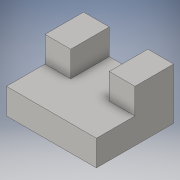
# Autodesk Inventor part: Figure 7_27_4
Saved by Autodesk Inventor 2016 (Build 200138000, 138)
## iProperties
Created: 2016-07-18
Part Number: Figure 7_27_4
Material: Generic
Document SubType Name: Modeling
Designer: cfkguest
Density: 1 g/cm^3
Appearance: Default
Author: cfkguest
Autodesk Inventor part; units mm, degrees
ref_plane "YZ Plane" through (0, 0, 0) normal (1, 0, 0) x (0, 1, 0)
ref_plane "XZ Plane" through (0, 0, 0) normal (0, 1, 0) x (-1, 0, 0)
ref_plane "XY Plane" through (0, 0, 0) normal (0, 0, 1) x (1, 0, 0)
sketch "Sketch1" plane through (0, 0, 0) normal (0, 0, 1) x (1, 0, 0)
  line L0 (-24.7144, 9.5678) -> (19.7356, 9.5678)
  line L1 (19.7356, 9.5678) -> (19.7356, -15.8322)
  line L2 (19.7356, -15.8322) -> (-24.7144, -15.8322)
  line L3 (-24.7144, -15.8322) -> (-24.7144, 9.5678)
  point P0 (0, 0)
  dimension "d0" = 44.45
  dimension "d1" = 25.4
  constraints: 8 end point, 2 parallel, 1 horizontal, 1 perpendicular
  measures "d0" distance of L0.start L0.end
  measures "d1" distance of L2.end L0.start
extrude "Extrusion1" add sketch "Sketch1" along normal blind 38.1
sketch "Sketch2" plane through (-24.7144, 9.5678, 0) normal (0, 1, 0) x (1, 0, 0)
  line L0 (0, 0) -> (0, -38.1) projected
  line L1 (44.45, 0) -> (44.45, -38.1) projected
  line L2 (0, -19.05) -> (44.45, -19.05)
  line L3 (44.45, -19.05) -> (44.45, -38.1)
  line L4 (44.45, -38.1) -> (0, -38.1)
  line L5 (0, -38.1) -> (0, -19.05)
  line L6 (0, 0) -> (44.45, 0) projected
  point P0 (24.7144, 0)
  dimension "d4" = 19.05
  constraints: 8 end point, 2 parallel, 1 horizontal, 1 midpoint, 1 perpendicular
  measures "d4" distance between parallel lines of L6 L2
extrude "Extrusion2" cut sketch "Sketch2" against normal blind 12.7 contours L2 L1 L4 L0
sketch "Sketch3" plane through (-24.7144, 9.5678, 0) normal (0, 1, 0) x (1, 0, 0)
  line L0 (0, -19.05) -> (44.45, -19.05) projected
  line L1 (12.7, -19.05) -> (31.75, -19.05)
  line L2 (31.75, -19.05) -> (31.75, 0)
  line L3 (31.75, 0) -> (12.7, 0)
  line L4 (12.7, 0) -> (12.7, -19.05)
  line L5 (0, 0) -> (0, -19.05) projected
  line L6 (44.45, 0) -> (44.45, -19.05) projected
  point P0 (24.7144, 0)
  dimension "d7" = 12.7
  dimension "d8" = 12.7
  dimension "d9" = 19.05
  constraints: 8 end point, 2 parallel, 1 horizontal, 1 perpendicular, 1 point on line
  measures "d7" distance between parallel lines of L5 L4
  measures "d8" distance between parallel lines of L6 L2
  measures "d9" distance of L3.end L1.start
extrude "Extrusion3" cut sketch "Sketch3" against normal blind 12.7
body "Solid1"
